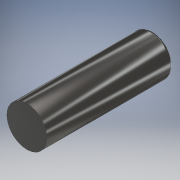
# Autodesk Inventor part: モーター100：1軸
Saved by Autodesk Inventor 2018 (Build 220112000, 112)
## iProperties
Part Number: モーター100：1軸
Material: 一般
Document SubType Name: Modeling
Designer: eieio
Density: 1 g/cm^3
Appearance: 鋼材 メッキ
Author: eieio
Autodesk Inventor part; units mm, degrees
ref_plane "YZ Plane" through (0, 0, 0) normal (1, 0, 0) x (0, 1, 0)
ref_plane "XZ Plane" through (0, 0, 0) normal (0, 1, 0) x (-1, 0, 0)
ref_plane "XY Plane" through (0, 0, 0) normal (0, 0, 1) x (1, 0, 0)
sketch "スケッチ1" plane through (0, 0, 0) normal (0, 1, 0) x (-1, 0, 0)
  circle A0 centre (0, 0) radius 3
  dimension "d0" = 6
  constraints: 1 centre point, 1 coincident
  measures "d0" diameter of A0
extrude "押し出し1" add sketch "スケッチ1" along normal blind 4
sketch "スケッチ2" plane through (0, 4, 0) normal (0, 1, 0) x (1, 0, 0)
  circle A0 centre (0, 0) radius 3 projected
  line L0 (0, 3) -> (0, 2)
  line L1 (0, 2) -> (2.2361, 2)
  arc A1 (-2.2361, 2) -> (2.2361, 2) centre (0, 0) ccw
  line L2 (-2.2361, 2) -> (0, 2)
  dimension "d3" = 1
  constraints: 6 end point, 6 point on circle, 1 centre point, 1 coincident, 1 horizontal, 1 vertical
  measures "d3" distance of L0.start L0.end
extrude "押し出し2" add sketch "スケッチ2" along normal blind 12 contours A0 L2 L1
sketch "スケッチ3" plane through (0, 0, 0) normal (0, -1, 0) x (1, 0, 0)
  circle A0 centre (0, 0) radius 3
  constraints: 1 centre point, 1 coincident
extrude "押し出し3" add sketch "スケッチ3" along normal blind 3
fillet "フィレット1" radius 0.4 1 edges at (0, 16, 3)
